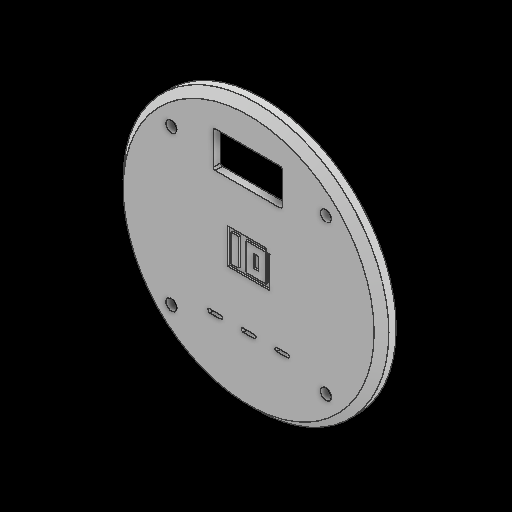
# Autodesk Inventor part: WheelEncoderCover
Saved by Autodesk Inventor 2025.2 (Build 292293000, 293)
## iProperties
Created: 2026-02-04
Part Number: WheelEncoderCover
Material: Generic
Document SubType Name: Modeling
Designer: valer
Density: 1 g/cm^3
Appearance: Default
Author: valer
Autodesk Inventor part; units mm, degrees
ref_plane "YZ Plane" through (0, 0, 0) normal (1, 0, 0) x (0, 1, 0)
ref_plane "XZ Plane" through (0, 0, 0) normal (0, 1, 0) x (-1, 0, 0)
ref_plane "XY Plane" through (0, 0, 0) normal (0, 0, 1) x (1, 0, 0)
sketch "Base" plane through (0, 0, 0) normal (0, 0, 1) x (1, 0, 0)
  circle A0 centre (0, 0) radius 36.125
  circle A1 centre (0, 0) radius 33.125
  circle A2 centre (0, 0) radius 34.625 construction
  dimension "d1" = 66.25
  dimension "d2" = 3
  dimension "d3" = 1.5
  constraints: 3 centre point, 3 coincident
  measures "d1" diameter of A1
  measures "d2" radial gap between concentric circles of A0 A1
  measures "d3" radial gap between concentric circles of A0 A2
extrude "BaseFeature" add sketch "Base" along normal blind 2
sketch "Cap" plane through (0, 0, 2) normal (0, 0, 1) x (1, 0, 0)
  circle A0 centre (0, 0) radius 36.125 projected
extrude "CapFeature" add sketch "Cap" along normal blind 2
chamfer "CapChamferFeature" distance 2 angle 45 1 edges at (-36.125, 0, 4)
sketch "MountHoles" plane through (0, 0, 4) normal (0, 0, 1) x (1, 0, 0)
  circle A0 centre (-20.9919, -21) radius 1.25 projected
  circle A1 centre (-20.9919, 21) radius 1.25 projected
  circle A2 centre (21.0081, -21) radius 1.25 projected
  circle A3 centre (21.0081, 21) radius 1.25 projected
hole "MountHolesFeature" at (-20.9919, -21, 4) at (-20.9919, 21, 4) at (21.0081, 21, 4) at (21.0081, -21, 4) direction (0, 0, -1) diameter 3 end through all
sketch "CapHoles" plane through (0, 0, 4) normal (0, 0, 1) x (1, 0, 0)
  line L0 (-7.125, -17.7082) -> (-11.125, -17.7082) projected
  line L1 (-11.125, -17.7082) -> (-11.125, -16.7082) projected
  line L2 (-7.125, -16.7082) -> (-7.125, -17.7082) projected
  line L3 (-11.125, -16.7082) -> (-7.125, -16.7082) projected
  line L4 (-2, -17.7082) -> (-2, -16.7082) projected
  line L5 (2, -17.7082) -> (-2, -17.7082) projected
  line L6 (-2, -16.7082) -> (2, -16.7082) projected
  line L7 (2, -16.7082) -> (2, -17.7082) projected
  line L8 (7.125, -17.7082) -> (7.125, -16.7082) projected
  line L9 (11.125, -17.7082) -> (7.125, -17.7082) projected
  line L10 (7.125, -16.7082) -> (11.125, -16.7082) projected
  line L11 (11.125, -16.7082) -> (11.125, -17.7082) projected
  line L12 (-9.125, 25.943) -> (-9.125, 17.093) construction
  line L13 (8.695, 17.093) -> (8.695, 25.943) construction
  line L14 (-9.125, 25.943) -> (8.695, 25.943) construction
  line L15 (-9.125, 17.093) -> (8.695, 17.093) construction
  line L16 (-9.625, 16.593) -> (-9.625, 26.443)
  line L17 (-9.625, 26.443) -> (9.195, 26.443)
  line L18 (9.195, 26.443) -> (9.195, 16.593)
  line L19 (9.195, 16.593) -> (-9.625, 16.593)
  point P0 (0, 0)
  dimension "d22" = 0.5
  constraints: 12 end point, 2 parallel, 1 horizontal, 3 other
  measures "d22" distance between parallel lines of L12 L16
extrude "CapHolesFeature" cut sketch "CapHoles" against normal through all
fillet "CapHoleFilletsFeature" radius 0.5 16 edges at (-9.625, 26.443, 3) (-9.625, 16.593, 3) (9.195, 26.443, 3) (9.195, 16.593, 3) (-11.125, -16.7082, 3) (-11.125, -17.7082, 3) (-7.125, -16.7082, 3) (-7.125, -17.7082, 3) (-2, -17.7082, 3) (-2, -16.7082, 3) (2, -17.7082, 3) (2, -16.7082, 3) (7.125, -17.7082, 3) (7.125, -16.7082, 3) (11.125, -17.7082, 3) (11.125, -16.7082, 3)
sketch "Logo" plane through (0, 0, 4) normal (0, 0, 1) x (1, 0, 0)
  line L0 (13.0396, 4.25) -> (13.0396, 5.25) construction
  line L1 (12.0396, 4.25) -> (13.0396, 4.25) construction
  line L2 (16.5396, 2.25) -> (15.0396, 2.25) construction
  line L3 (13.0396, 4.25) -> (18.5396, 4.25) construction
  line L4 (15.0396, -1.25) -> (16.5396, -1.25) construction
  line L5 (16.5396, -1.25) -> (16.5396, 2.25) construction
  line L6 (13.0396, -3.25) -> (13.0396, 4.25) construction
  line L7 (12.0396, 4.25) -> (12.0396, -4.25) construction
  line L8 (18.5396, -3.25) -> (13.0396, -3.25) construction
  line L9 (18.5396, 4.25) -> (18.5396, -3.25) construction
  line L10 (23.5396, 5.25) -> (13.0396, 5.25) construction
  line L11 (22.5396, 4.25) -> (20.5396, 4.25) construction
  line L12 (20.5396, 4.25) -> (20.5396, -3.25) construction
  line L13 (20.5396, -3.25) -> (22.5396, -3.25) construction
  line L14 (22.5396, -3.25) -> (22.5396, 4.25) construction
  line L15 (15.0396, 2.25) -> (15.0396, -1.25) construction
  line L16 (0, -54.0958) -> (0, 56.5932) construction
  line L17 (12.0396, -4.25) -> (23.5396, -4.25) construction
  line L18 (23.5396, -4.25) -> (23.5396, 5.25) construction
  line L19 (-50.575, 0) -> (50.575, 0) construction
  line L20 (8.8948, -38.2831) -> (8.8948, 40.7805) construction
  line L21 (1.25, 2.25) -> (2.75, 2.25)
  line L22 (4.75, 4.25) -> (-0.75, 4.25)
  line L23 (2.75, 2.25) -> (2.75, -1.25)
  line L24 (1.25, -1.25) -> (1.25, 2.25)
  line L25 (2.75, -1.25) -> (1.25, -1.25)
  line L26 (-5.75, 5.25) -> (4.75, 5.25)
  line L27 (-0.75, -3.25) -> (4.75, -3.25)
  line L28 (4.75, 4.25) -> (4.75, 5.25)
  line L29 (-2.75, -3.25) -> (-4.75, -3.25)
  line L30 (-0.75, 4.25) -> (-0.75, -3.25)
  line L31 (-4.75, -3.25) -> (-4.75, 4.25)
  line L32 (-4.75, 4.25) -> (-2.75, 4.25)
  line L33 (-2.75, 4.25) -> (-2.75, -3.25)
  line L34 (4.75, -3.25) -> (4.75, 4.25)
  line L35 (5.75, 4.25) -> (4.75, 4.25)
  line L36 (5.75, 4.25) -> (5.75, -4.25)
  line L37 (5.75, -4.25) -> (-5.75, -4.25)
  line L38 (-5.75, -4.25) -> (-5.75, 5.25)
  point P0 (0, 0)
  point P1 (21.5396, -3.25)
  point P2 (17.7896, -4.25)
  point P3 (12.0396, 0)
  point P4 (-3.75, -3.25)
  point P5 (0, -4.25)
  point P6 (5.75, 0)
  point P7 (0, -4.25)
  dimension "d27" = 1.5
  dimension "d28" = 1
  dimension "d29" = 1
  dimension "d31" = 2
  dimension "d32" = 2
  dimension "d33" = 2
  dimension "d34" = 2
  dimension "d35" = 8.5
  dimension "d39" = 1
  dimension "d40" = 1
  dimension "d42" = 2
  dimension "d43" = 3.5
  dimension "d46" = 1
  dimension "d47" = 2
  dimension "d48" = 1
  dimension "d49" = 1
  dimension "d50" = 1
  dimension "d51" = 1
  constraints: 74 end point, 20 symmetric about line, 7 parallel, 4 midpoint, 4 perpendicular, 2 collinear, 2 point on line, 2 vertical, 1 horizontal
  measures "d27" distance between parallel lines of L15 L5
  measures "d28" distance between parallel lines of L7 L6
  measures "d29" distance between parallel lines of L10 L3
  measures "d31" distance between parallel lines of L12 L9
  measures "d32" distance between parallel lines of L12 L14
  measures "d33" distance between parallel lines of L5 L9
  measures "d34" distance between parallel lines of L6 L15
  measures "d35" distance of L1.start L7.end
  measures "d39" distance of L3.start L10.end
  measures "d40" distance of L1.start L3.start
  measures "d42" distance between parallel lines of L8 L4
  measures "d43" distance of L2.end L15.end
  measures "d46" distance between parallel lines of L10 L11
  measures "d47" distance between parallel lines of L3 L2
  measures "d48" distance between parallel lines of L8 L17
  measures "d49" distance from line of point (21.54, -3.25) L17
  measures "d50" distance between parallel lines of L18 L14
  measures "d51" distance between parallel lines of L13 L17
extrude "LogoFeature" cut sketch "Logo" against normal blind 0.5
equation "\"d3\" = 0.5 * d2"
body "Solid1"
